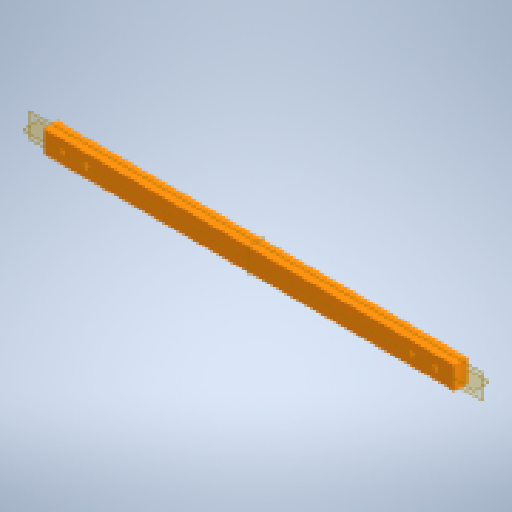
# Autodesk Inventor part: conector_eixos_001
Saved by Autodesk Inventor 2026 (Build 300175000, 175)
## iProperties
Created: 2025-11-27
Part Number: conector_eixos_001
Material: ABS Plastic
Document SubType Name: Modeling
Designer: Carlos Dias
Density: 1.06 g/cm^3
Appearance: Orange
Author: Carlos Dias
Autodesk Inventor part; units mm, degrees
sketch "Sketch1" plane through (0, 0, 0) normal (0, 0, 1) x (1, 0, 0)
  line L0 (-120, 6.5) -> (120, 6.5)
  line L1 (120, 6.5) -> (120, -6.5)
  line L2 (120, -6.5) -> (-120, -6.5)
  line L3 (-120, -6.5) -> (-120, 6.5)
  line L4 (-120, 6.5) -> (120, -6.5) construction
  line L5 (120, 6.5) -> (-120, -6.5) construction
  point P0 (0, 0)
  point P1 (0, 0)
  dimension "d0" = 240
  dimension "d1" = 13
  constraints: 12 end point, 2 midpoint, 2 parallel, 1 coincident, 1 horizontal, 1 perpendicular
  measures "d0" distance of L0.start L0.end
  measures "d1" distance of L0.end L1.end
extrude "Extrusion1" add sketch "Sketch1" along normal mid plane 8
sketch "Sketch2" plane through (0, 0, 4) normal (0, 0, 1) x (1, 0, 0)
  circle A0 centre (-109, 0) radius 1.5 projected
  circle A1 centre (-95, 0) radius 1.5 projected
  circle A2 centre (95, 0) radius 1.5 projected
  circle A3 centre (109, 0) radius 1.5 projected
  point P0 (0, 0)
extrude "Extrusion2" cut sketch "Sketch2" against normal through all
body "Solid1"
